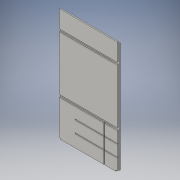
# Autodesk Inventor part: Left Side
Saved by Autodesk Inventor 2016 (Build 200138000, 138)
## iProperties
Created: 2017-10-30
Part Number: Left Side
Material: Generic
Document SubType Name: Modeling
Designer: mathaetaes
Density: 1 g/cm^3
Appearance: Default
Author: mathaetaes
Autodesk Inventor part; units mm, degrees
ref_plane "YZ Plane" through (0, 0, 0) normal (1, 0, 0) x (0, 1, 0)
ref_plane "XZ Plane" through (0, 0, 0) normal (0, 1, 0) x (-1, 0, 0)
ref_plane "XY Plane" through (0, 0, 0) normal (0, 0, 1) x (1, 0, 0)
sketch "Sketch1" plane through (0, 0, 0) normal (0, 0, 1) x (1, 0, 0)
  line L0 (-222.9556, 663.6813) -> (246.9444, 663.6813)
  line L1 (246.9444, 663.6813) -> (246.9444, -238.0187)
  line L2 (246.9444, -238.0187) -> (-222.9556, -238.0187)
  line L3 (-222.9556, -238.0187) -> (-222.9556, 663.6813)
  point P0 (0, 0)
  dimension "d0" = 469.9
  dimension "d1" = 901.7
  constraints: 8 end point, 2 parallel, 1 horizontal, 1 perpendicular
  measures "d0" distance of L1.end L2.end
  measures "d1" distance of L0.end L1.end
extrude "Board" add sketch "Sketch1" along normal blind 19.05
sketch "Sketch2" plane through (0, 0, 19.05) normal (0, 0, 1) x (1, 0, 0)
  line L0 (-222.9556, 663.6813) -> (-222.9556, -238.0187) projected
  line L1 (246.9444, -238.0187) -> (246.9444, 663.6813) projected
  line L2 (-222.9556, 69.9563) -> (246.9444, 69.9563)
  line L3 (246.9444, 69.9563) -> (246.9444, 50.9063)
  line L4 (246.9444, 50.9063) -> (-222.9556, 50.9063)
  line L5 (-222.9556, 50.9063) -> (-222.9556, 69.9563)
  line L6 (246.9444, 663.6813) -> (-222.9556, 663.6813) projected
  line L7 (-222.9556, -238.0187) -> (246.9444, -238.0187) projected
  point P0 (0, 0)
  dimension "d4" = 19.05
  dimension "d19" = 288.925
  constraints: 8 end point, 2 parallel, 2 point on line, 1 horizontal, 1 perpendicular
  measures "d4" distance between parallel lines of L4 L2
  measures "d19" distance between parallel lines of L7 L4
extrude "Inner Lower Shelf Dado" cut sketch "Sketch2" against normal blind 9.525 contours L2 L1 L4 L0
sketch "Sketch4" plane through (0, 0, 19.05) normal (0, 0, 1) x (1, 0, 0)
  line L0 (-222.9556, 523.9813) -> (246.9444, 523.9813)
  line L1 (246.9444, 523.9813) -> (246.9444, 504.9313)
  line L2 (246.9444, 504.9313) -> (-222.9556, 504.9313)
  line L3 (-222.9556, 504.9313) -> (-222.9556, 523.9813)
  line L4 (246.9444, 663.6813) -> (-222.9556, 663.6813) projected
  line L5 (246.9444, -238.0187) -> (246.9444, 663.6813) projected
  line L6 (-222.9556, 663.6813) -> (-222.9556, -238.0187) projected
  point P0 (0, 0)
  point P1 (246.9444, 69.9563)
  point P2 (-222.9556, 69.9563)
  dimension "d20" = 19.05
  dimension "d21" = 139.7
  constraints: 8 end point, 2 collinear, 2 parallel, 1 horizontal, 1 perpendicular
  measures "d20" distance of L0.end L1.end
  measures "d21" distance between parallel lines of L4 L0
extrude "Inner Upper Shelf Dado" cut sketch "Sketch4" against normal blind 9.525 contours L0 L1 L2 L3
sketch "Sketch7" plane through (0, 0, 0) normal (0, 0, -1) x (-1, 0, 0)
  line L0 (222.9556, 663.6813) -> (-246.9444, 663.6813) projected
  line L1 (-246.9444, 663.6813) -> (222.9556, 663.6813)
  line L2 (222.9556, 663.6813) -> (222.9556, 650.9813)
  line L3 (222.9556, 650.9813) -> (-246.9444, 650.9813)
  line L4 (-246.9444, 650.9813) -> (-246.9444, 663.6813)
  line L5 (222.9556, -238.0187) -> (222.9556, 663.6813) projected
  line L6 (-246.9444, -238.0187) -> (222.9556, -238.0187)
  line L7 (222.9556, -238.0187) -> (222.9556, -228.4937)
  line L8 (222.9556, -228.4937) -> (-246.9444, -228.4937)
  line L9 (-246.9444, -228.4937) -> (-246.9444, -238.0187)
  line L10 (-246.9444, -238.0187) -> (222.9556, -238.0187) projected
  point P0 (0, 0)
  dimension "d32" = 12.7
  dimension "d40" = 9.525
  constraints: 16 end point, 4 parallel, 3 collinear, 2 horizontal, 2 perpendicular
  measures "d32" distance of L1.end L2.end
  measures "d40" distance between parallel lines of L6 L8
extrude "Top and Bottom Exterior Dados" cut sketch "Sketch7" against normal blind 9.525
sketch "Sketch9" plane through (246.9444, -238.0187, 19.05) normal (1, 0, 0) x (0, 0, -1)
  line L0 (0, 901.7) -> (9.525, 901.7)
  line L1 (9.525, 901.7) -> (9.525, 0)
  line L2 (9.525, 0) -> (0, 0)
  line L3 (0, 0) -> (0, 901.7)
  line L4 (9.525, 901.7) -> (0, 901.7) projected
  line L5 (9.525, 0) -> (0, 0) projected
  line L6 (0, 0) -> (0, 742.95) projected
  point P0 (19.05, 238.0187)
  point P1 (0, 307.975)
  dimension "d41" = 9.525
  constraints: 8 end point, 3 collinear, 2 parallel, 1 horizontal, 1 perpendicular
  measures "d41" distance between parallel lines of L1 L3
extrude "Back Panel Notch" cut sketch "Sketch9" against normal blind 6.35
sketch "Sketch10" plane through (0, 0, 0) normal (0, 0, -1) x (-1, 0, 0)
  line L0 (-145.3444, 650.9813) -> (-107.2444, 650.9813)
  line L1 (-107.2444, 650.9813) -> (-107.2444, 630.3438)
  line L2 (-110.4194, 627.1688) -> (-142.1694, 627.1688)
  line L3 (-145.3444, 630.3438) -> (-145.3444, 650.9813)
  line L4 (-246.9444, 650.9813) -> (-246.9444, -228.4937) projected
  line L5 (222.9556, 650.9813) -> (-246.9444, 650.9813) projected
  line L6 (95.9556, 650.9813) -> (134.0556, 650.9813)
  line L7 (134.0556, 650.9813) -> (134.0556, 630.3438)
  line L8 (130.8806, 627.1688) -> (99.1306, 627.1688)
  line L9 (95.9556, 630.3438) -> (95.9556, 650.9813)
  arc A0 (-145.3444, 630.3438) -> (-142.1694, 627.1688) centre (-142.1694, 630.3438) ccw
  arc A1 (-110.4194, 627.1688) -> (-107.2444, 630.3438) centre (-110.4194, 630.3438) ccw
  arc A2 (95.9556, 630.3438) -> (99.1306, 627.1688) centre (99.1306, 630.3438) ccw
  arc A3 (130.8806, 627.1688) -> (134.0556, 630.3438) centre (130.8806, 630.3438) ccw
  point P0 (0, 0)
  point P1 (-107.2444, 627.1688)
  point P2 (-145.3444, 627.1688)
  point P3 (134.0556, 627.1688)
  point P4 (95.9556, 627.1688)
  dimension "d44" = 38.1
  dimension "d45" = 23.8125
  dimension "d46" = 101.6
  dimension "d47" = 38.1
  dimension "d48" = 23.8125
  dimension "d49" = 203.2
  dimension "d50" = 3.175
  constraints: 16 end point, 8 point on circle, 8 point on line, 8 tangent, 4 centre point, 4 parallel, 3 equal radius, 2 collinear, 2 horizontal, 2 perpendicular
  measures "d44" distance of point (-107.244, 627.169) point (-145.344, 627.169)
  measures "d45" distance of L0.end point (-107.244, 627.169)
  measures "d46" distance between parallel lines of L3 L4
  measures "d47" distance of point (134.056, 627.169) point (95.956, 627.169)
  measures "d48" distance of L6.end point (134.056, 627.169)
  measures "d49" distance between parallel lines of L9 L1
  measures "d50" radius of A0
extrude "Top Hinge Notches" cut sketch "Sketch10" against normal blind 3.175
sketch "Sketch12" plane through (-222.9556, -238.0187, 19.05) normal (-1, 0, 0) x (0, 0, 1)
  line L0 (-9.525, 9.525) -> (-9.525, 0) projected
  line L1 (0, 901.7) -> (0, 0) projected
  line L2 (-9.525, 0) -> (0, 0)
  line L3 (0, 0) -> (0, 9.525)
  line L4 (0, 9.525) -> (-9.525, 9.525)
  line L5 (-9.525, 9.525) -> (-9.525, 0)
  line L6 (-19.05, 9.525) -> (-9.525, 9.525) projected
  point P0 (-19.05, 238.0187)
  point P1 (0, 288.925)
  constraints: 8 end point, 2 parallel, 1 collinear, 1 horizontal, 1 perpendicular, 1 point on line
extrude "Front notch to cover dado" cut sketch "Sketch12" against normal blind 6.35
sketch "Sketch3" plane through (0, 0, 19.05) normal (0, 0, 1) x (1, 0, 0)
  line L0 (240.5944, -133.2437) -> (-95.9556, -133.2437)
  line L1 (-95.9556, -133.2437) -> (-95.9556, -139.5937)
  line L2 (-95.9556, -139.5937) -> (240.5944, -139.5937)
  line L3 (240.5944, -139.5937) -> (240.5944, -133.2437)
  line L4 (-222.9556, -238.0187) -> (246.9444, -238.0187) projected
  line L5 (259.6444, -37.9937) -> (-95.9556, -37.9937)
  line L6 (-95.9556, -37.9937) -> (-95.9556, -44.3437)
  line L7 (-95.9556, -44.3437) -> (259.6444, -44.3437)
  line L8 (259.6444, -44.3437) -> (259.6444, -37.9937)
  line L9 (-222.9556, 663.6813) -> (-222.9556, -238.0187) projected
  line L10 (246.9444, 50.9063) -> (-222.9556, 50.9063) projected
  line L11 (246.9444, -228.4937) -> (240.5944, -228.4937) projected
  point P0 (0, 0)
  dimension "d9" = 6.35
  dimension "d14" = 6.35
  dimension "d17" = 88.9
  dimension "d26" = 127
  dimension "d67" = 88.9
  constraints: 16 end point, 4 parallel, 2 horizontal, 2 perpendicular, 1 collinear
  measures "d9" distance of L0.end L1.end
  measures "d14" distance of L5.end L6.end
  measures "d17" distance between parallel lines of L7 L0
  measures "d26" distance between parallel lines of L9 L6
  measures "d67" distance between parallel lines of L11 L2
extrude "Inner Wine Rack Dados" cut sketch "Sketch3" against normal blind 6.35
sketch "Sketch8" plane through (0, 0, 19.05) normal (0, 0, 1) x (1, 0, 0)
  line L0 (246.9444, 50.9063) -> (-222.9556, 50.9063) projected
  line L1 (132.6444, -238.0187) -> (138.9944, -238.0187)
  line L2 (138.9944, -238.0187) -> (138.9944, 50.9063)
  line L3 (138.9944, 50.9063) -> (132.6444, 50.9063)
  line L4 (132.6444, 50.9063) -> (132.6444, -238.0187)
  line L5 (-95.9556, -139.5937) -> (-95.9556, -133.2437) projected
  line L6 (-222.9556, -238.0187) -> (246.9444, -238.0187) projected
  point P0 (0, 0)
  dimension "d35" = 6.35
  dimension "d36" = 228.6
  constraints: 8 end point, 2 parallel, 1 collinear, 1 horizontal, 1 perpendicular, 1 point on line
  measures "d35" distance of L1.start L1.end
  measures "d36" distance between parallel lines of L5 L4
extrude "Vertical Wine Bottle False Back" cut sketch "Sketch8" against normal blind 9.525
sketch "Sketch13" plane through (0, 0, 9.525) normal (0, 0, -1) x (-1, 0, 0)
  line L0 (-246.9444, 650.9813) -> (-246.9444, -228.4937) projected
  line L1 (216.6056, -238.0187) -> (-240.5944, -238.0187) projected
  line L2 (-246.9444, -228.4937) -> (-227.8944, -228.4937)
  line L3 (-227.8944, -228.4937) -> (-227.8944, -238.0187)
  line L4 (-227.8944, -238.0187) -> (-246.9444, -238.0187)
  line L5 (-246.9444, -238.0187) -> (-246.9444, -228.4937)
  point P0 (0, 0)
  point P1 (-138.9944, -238.0187)
  dimension "d64" = 19.05
  constraints: 8 end point, 2 parallel, 1 horizontal, 1 perpendicular, 1 point on line
  measures "d64" distance of L3.end L4.end
extrude "Rear notch for bottom runner" cut sketch "Sketch13" against normal blind 19.05
equation "\"d6\" = 0.5 * d2"
equation "\"d22\" = 0.5 * d2"
equation "\"d47\" = d44"
equation "\"d48\" = d45"
equation "\"d49\" = 2 * d46"
equation "\"d37\" = 0.5 * d2"
equation "\"d2\" = 19.05"
body "Solid1"
